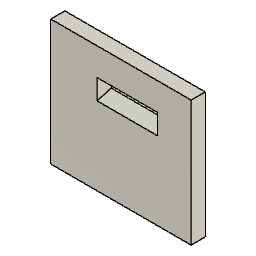
smartie_feed (Autodesk Fusion 360 design; units mm, degrees)
Autodesk Fusion 360 part; units mm, degrees
sketch "Smartie Feed" plane through (0, 0, 0) normal (0, 0, 1) x (1, 0, 0)
  line L0 (0, 0) -> (209, 0)
  line L1 (209, 0) -> (209, 21)
  line L2 (209, 21) -> (0, 21)
  line L3 (0, 21) -> (0, 0)
  dimension "d1" = 209
  dimension "d2" = 21
  constraint horizontal L0
  constraint vertical L1
  constraint horizontal L2
  constraint vertical L3
  constraint coincident L0.start L3.end
  measures "d1" distance of L0.start L0.end
  measures "d2" distance of L0.end L1.end
extrude "Extrude1" add sketch "Smartie Feed" along normal blind 187
sketch "Outlet" plane through (0, 0, 0) normal (0, -1, 0) x (1, 0, 0)
  line L0 (0, 0) -> (209, 0)
  line L1 (209, 0) -> (209, 187)
  line L2 (209, 187) -> (0, 187)
  line L3 (0, 187) -> (0, 0)
  line L4 (69, 146) -> (159, 146)
  line L5 (159, 146) -> (159, 116)
  line L6 (159, 116) -> (69, 116)
  line L7 (69, 116) -> (69, 146)
  dimension "d31" = 30
  dimension "d32" = 90
  dimension "d33" = 69
  dimension "d34" = 50
  dimension "d35" = 41
  constraint horizontal L4
  constraint vertical L5
  constraint horizontal L6
  constraint vertical L7
  measures "d31" distance of L4.end L5.end
  measures "d32" distance of L4.start L4.end
  measures "d33" distance of L3 L7
  measures "d34" distance of L1 L5
  measures "d35" distance of L2 L4
sketch "Inlet" plane through (0, 21, 0) normal (0, 1, 0) x (-1, 0, 0)
  line L0 (-209, 0) -> (0, 0)
  line L1 (0, 0) -> (0, 187)
  line L2 (0, 187) -> (-209, 187)
  line L3 (-209, 187) -> (-209, 0)
  line L4 (-69, 152) -> (-159, 152)
  line L5 (-159, 152) -> (-159, 122)
  line L6 (-159, 122) -> (-69, 122)
  line L7 (-69, 122) -> (-69, 152)
  dimension "d36" = 90
  dimension "d37" = 69
  dimension "d38" = 30
  dimension "d39" = 35
  dimension "d40" = 50
  constraint horizontal L4
  constraint vertical L5
  constraint horizontal L6
  constraint vertical L7
  measures "d36" distance of L4.start L4.end
  measures "d37" distance of L1 L7
  measures "d38" distance of L4.start L6.end
  measures "d39" distance of L2 L4
  measures "d40" distance of L3 L5
loft "Loft9" cut profiles "Inlet", "Outlet" section 1 contours L4 L5 L6 L7 section 2 contours L4 L5 L6 L7
sketch "Sketch6" plane through (0, 21, 0) normal (0, 1, 0) x (-1, 0, 0)
  line L0 (-69, 152) -> (-69, 122)
  line L1 (-69, 122) -> (-159, 122)
  line L2 (-159, 122) -> (-159, 152)
  line L3 (-159, 152) -> (-69, 152)
  line L4 (-209, 0) -> (0, 0)
  line L5 (0, 0) -> (0, 187)
  line L6 (0, 187) -> (-209, 187)
  line L7 (-209, 187) -> (-209, 0)
  circle A0 centre (-164, 172) radius 2.75
  circle A1 centre (-64, 172) radius 2.75
  circle A2 centre (-164, 102) radius 2.75
  circle A3 centre (-64, 102) radius 2.75
  dimension "d43" = 5.5
  dimension "d44" = 5.5
  dimension "d45" = 5.5
  dimension "d46" = 5.5
  dimension "d49" = 64
  dimension "d50" = 64
  dimension "d51" = 164
  dimension "d52" = 164
  dimension "d53" = 20
  dimension "d54" = 20
  dimension "d55" = 20
  dimension "d56" = 20
  measures "d43" diameter of A0
  measures "d44" diameter of A2
  measures "d45" diameter of A1
  measures "d46" diameter of A3
  measures "d49" distance of L5 A1.centre
  measures "d50" distance of L5 A3.centre
  measures "d51" distance of L5 A0.centre
  measures "d52" distance of L5 A2.centre
  measures "d53" distance of L3 A1.centre
  measures "d54" distance of L3 A0.centre
  measures "d55" distance of L1 A2.centre
  measures "d56" distance of L1 A3.centre
extrude "Extrude2" cut sketch "Sketch6" against normal blind 1.5 contours A0 | A1 | A2 | A3
equation "d1 = 219 mm - 10 mm"
equation "d3 = 166 mm + 21 mm"
equation "outletHeight = 15 mm" comment "Height of the outlets into the sorted containers"
equation "outletWidth = 20 mm" comment "Width of the outlets into the sorted containers"
equation "sortedContainersMidpointWidth = sortedContainersWidth + polycarbonateThickness" comment "Width between the midpoints of the sorted containers"
equation "sortedContainersWidth = 60 mm" comment "Width of the sorted containers"
equation "sortedContainersHeight = 113 mm" comment "Height of the sorted containers"
equation "polycarbonateThickness = 6 mm" comment "Thickness of the polycarbonate"
equation "sortedContainersMidpointHeight = sortedContainersHeight + polycarbonateThickness" comment "Height between the midpoints of the sorted containers"
equation "d33 = 90 mm - 21 mm"
equation "d35 = 30 mm - 21 mm + 5 mm + 6 mm + 21 mm"
equation "d37 = 90 mm - 21 mm"
equation "d39 = 30 mm - 21 mm + 5 mm + 21 mm"
equation "magnetDiameter = 5 mm"
equation "magnetHeight = 1.5 mm"
equation "d43 = magnetDiameter + 0.5 mm"
equation "d44 = magnetDiameter + 0.5 mm"
equation "d45 = magnetDiameter + 0.5 mm"
equation "d46 = magnetDiameter + 0.5 mm"
equation "d47 = -magnetHeight"
equation "d49 = 75 mm - 21 mm + 10 mm"
equation "d50 = 75 mm - 21 mm + 10 mm"
equation "d51 = 195 mm - 10 mm - 21 mm"
equation "d52 = 195 mm - 10 mm - 21 mm"
named bodies: "Smartie Feed"
